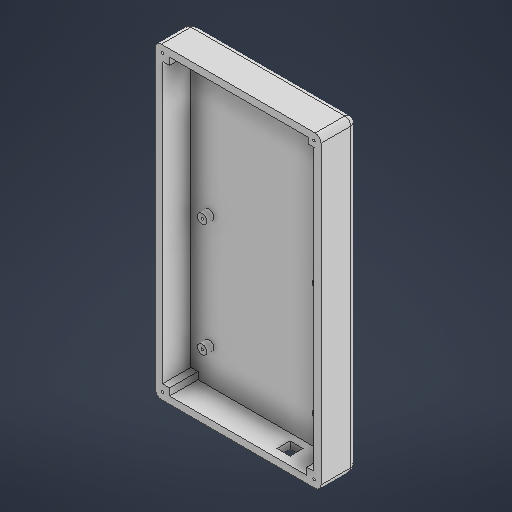
# Autodesk Inventor part: Bottom_Shell
Saved by Autodesk Inventor 2026.2 (Build 302298010, 298A)
## iProperties
Created: 2026-03-03
Part Number: Bottom_Shell
Material: Generic
Document SubType Name: Modeling
Designer: kjedr
Density: 1 g/cm^3
Appearance: Default
Author: kjedr
Autodesk Inventor part; units mm, degrees
ref_plane "YZ Plane" through (0, 0, 0) normal (1, 0, 0) x (0, 1, 0)
ref_plane "XZ Plane" through (0, 0, 0) normal (0, 1, 0) x (-1, 0, 0)
ref_plane "XY Plane" through (0, 0, 0) normal (0, 0, 1) x (1, 0, 0)
sketch "Sketch1" plane through (0, 0, 0) normal (0, 0, 1) x (1, 0, 0)
  line L0 (0, 0) -> (88.9, 0)
  line L1 (88.9, 0) -> (88.9, 165.1)
  line L2 (88.9, 165.1) -> (0, 165.1)
  line L3 (0, 165.1) -> (0, 0)
  dimension "d0" = 88.9
  dimension "d1" = 165.1
  constraints: 8 end point, 2 parallel, 1 horizontal, 1 perpendicular
  measures "d0" distance of L2.end L1.end
  measures "d1" distance of L1.end L0.end
extrude "Extrusion1" add sketch "Sketch1" along normal blind 19.05
sketch "Sketch2" plane through (0, 0, 19.05) normal (0, 0, 1) x (1, 0, 0)
  line L0 (3.81, 3.81) -> (85.09, 3.81)
  line L1 (85.09, 3.81) -> (85.09, 161.29)
  line L2 (85.09, 161.29) -> (3.81, 161.29)
  line L3 (3.81, 161.29) -> (3.81, 3.81)
  line L4 (0, 165.1) -> (0, 0) projected
  line L5 (0, 0) -> (88.9, 0) projected
  line L6 (88.9, 0) -> (88.9, 165.1) projected
  line L7 (88.9, 165.1) -> (0, 165.1) projected
  point P0 (88.9, 82.55)
  dimension "d4" = 3.81
  dimension "d5" = 3.81
  dimension "d6" = 3.81
  dimension "d7" = 3.81
  constraints: 8 end point, 2 parallel, 1 horizontal, 1 midpoint, 1 perpendicular
  measures "d4" distance between parallel lines of L4 L3
  measures "d5" distance between parallel lines of L5 L0
  measures "d6" distance from line of point (88.9, 82.55) L1
  measures "d7" distance between parallel lines of L7 L2
extrude "Extrusion2" cut sketch "Sketch2" against normal blind 15.24 contours L3 L2 L1 L0
fillet "Fillet1" radius 3.175 8 edges at (44.45, 165.1, 0) (88.9, 82.55, 0) (88.9, 0, 9.525) (0, 82.55, 0) (44.45, 0, 0) (88.9, 165.1, 9.525) (0, 165.1, 9.525) (0, 0, 9.525)
sketch "Sketch6" plane through (0, 0, 3.81) normal (0, 0, 1) x (1, 0, 0)
  line L0 (9.181, 90.81) -> (79.719, 90.81) construction
  line L1 (79.719, 90.81) -> (79.719, 6.81) construction
  line L2 (79.719, 6.81) -> (9.181, 6.81) construction
  line L3 (9.181, 6.81) -> (9.181, 90.81) construction
  circle A0 centre (13.6528, 83.516) radius 1.6 construction
  circle A1 centre (75.2732, 83.516) radius 1.6 construction
  circle A2 centre (13.6528, 22.81) radius 1.6 construction
  circle A3 centre (75.2732, 22.81) radius 1.6 construction
  line L4 (3.81, 161.29) -> (85.09, 161.29) projected
  line L5 (3.175, 0) -> (85.725, 0) projected
  line L6 (85.09, 3.81) -> (3.81, 3.81) projected
  circle A4 centre (13.6528, 83.516) radius 2.54
  circle A5 centre (75.2732, 83.516) radius 2.54
  circle A6 centre (13.6528, 22.81) radius 2.54
  circle A7 centre (75.2732, 22.81) radius 2.54
  point P0 (0, 0)
  point P1 (44.45, 90.81)
  point P2 (44.45, 161.29)
  point P3 (18.161, 33.81)
  point P4 (50.719, 19.31)
  point P5 (64.296, 6.81)
  dimension "d18" = 70.538
  dimension "d19" = 84
  dimension "d30" = 3.2
  dimension "d31" = 60.706
  dimension "d32" = 61.6204
  dimension "d33" = 16
  dimension "d34" = 4.4458
  dimension "d36" = 3
  dimension "d37" = 27
  dimension "d38" = 8.98
  dimension "d39" = 12.5
  dimension "d40" = 29
  dimension "d41" = 15.423
  dimension "d69" = 5.08
  dimension "d70" = 5.08
  dimension "d71" = 5.08
  dimension "d72" = 5.08
  constraints: 8 centre point, 8 end point, 4 coincident, 3 equal radius, 3 vertical alignment, 2 horizontal alignment, 2 midpoint, 2 parallel, 1 horizontal, 1 perpendicular, 1 point on line
  measures "d18" distance of L1.end L2.end
  measures "d19" distance of L0.end L1.end
  measures "d30" diameter of A0
  measures "d31" distance of A2.centre A0.centre
  measures "d32" distance of A3.centre A2.centre
  measures "d33" distance from line of L2 A3.centre
  measures "d34" distance from line of L1 A3.centre
  measures "d36" distance between parallel lines of L6 L2
  measures "d37" distance from line of L2 point (18.161, 33.81)
  measures "d38" distance from line of L3 point (18.161, 33.81)
  measures "d39" distance from line of L2 point (50.719, 19.31)
  measures "d40" distance from line of L1 point (50.719, 19.31)
  measures "d41" distance from line of L1 point (64.296, 6.81)
  measures "d69" diameter of A4
  measures "d70" diameter of A5
  measures "d71" diameter of A6
  measures "d72" diameter of A7
sketch "Sketch11" plane through (3.175, 0, 3.175) normal (0, -1, 0) x (1, 0, 0)
  line L0 (85.725, 0) -> (85.725, 15.875) projected
  line L1 (57.6124, 11.4375) -> (64.6124, 11.4375)
  line L2 (64.6124, 11.4375) -> (64.6124, 4.4375)
  line L3 (64.6124, 4.4375) -> (57.6124, 4.4375)
  line L4 (57.6124, 4.4375) -> (57.6124, 11.4375)
  line L5 (57.6124, 11.4375) -> (64.6124, 4.4375) construction
  line L6 (64.6124, 11.4375) -> (57.6124, 4.4375) construction
  line L7 (82.55, 15.875) -> (82.55, 0) projected
  line L8 (0, 15.875) -> (82.55, 15.875) projected
  point P0 (-3.175, -3.175)
  point P1 (61.1124, 7.9375)
  point P2 (64.6124, 7.9375)
  point P3 (82.55, 7.9375)
  point P4 (41.275, 15.875)
  dimension "d43" = 7
  dimension "d44" = 7
  dimension "d68" = 19.8374
  constraints: 12 end point, 5 midpoint, 2 parallel, 1 horizontal, 1 horizontal alignment, 1 perpendicular
  measures "d43" distance of L2.end L3.end
  measures "d44" distance of L1.end L2.end
  measures "d68" horizontal distance of point (41.275, 15.875) point (61.112, 7.938)
extrude "Extrusion5" cut sketch "Sketch11" against normal up to surface (3.81 mm away)
sketch "Sketch12" plane through (0, 0, 3.81) normal (0, 0, 1) x (1, 0, 0)
  line L0 (3.81, 3.81) -> (3.81, 161.29) projected
  line L1 (3.81, 3.81) -> (7.62, 3.81)
  line L2 (7.62, 3.81) -> (7.62, 7.62)
  line L3 (7.62, 7.62) -> (3.81, 7.62)
  line L4 (3.81, 7.62) -> (3.81, 3.81)
  line L5 (3.81, 161.29) -> (85.09, 161.29) projected
  line L6 (3.81, 161.29) -> (7.62, 161.29)
  line L7 (7.62, 161.29) -> (7.62, 157.48)
  line L8 (7.62, 157.48) -> (3.81, 157.48)
  line L9 (3.81, 157.48) -> (3.81, 161.29)
  arc A0 (88.9, 161.925) -> (85.725, 165.1) centre (85.725, 161.925) ccw projected
  line L10 (85.725, 161.925) -> (81.915, 161.925)
  line L11 (81.915, 161.925) -> (81.915, 158.115)
  line L12 (81.915, 158.115) -> (85.725, 158.115)
  line L13 (85.725, 158.115) -> (85.725, 161.925)
  line L14 (85.09, 161.29) -> (85.09, 3.81) projected
  line L15 (85.09, 3.81) -> (81.28, 3.81)
  line L16 (81.28, 3.81) -> (81.28, 7.62)
  line L17 (81.28, 7.62) -> (85.09, 7.62)
  line L18 (85.09, 7.62) -> (85.09, 3.81)
  point P0 (0, 0)
  point P1 (85.09, 158.115)
  point P2 (81.915, 161.29)
  dimension "d47" = 3.81
  dimension "d48" = 3.81
  dimension "d49" = 3.81
  dimension "d50" = 3.81
  dimension "d51" = 3.81
  dimension "d52" = 3.81
  dimension "d53" = 3.81
  dimension "d54" = 3.81
  constraints: 32 end point, 8 parallel, 4 horizontal, 4 perpendicular
  measures "d47" distance of L3.end L2.end
  measures "d48" distance of L2.end L1.end
  measures "d49" distance of L7.end L8.end
  measures "d50" distance of L12.end L11.end
  measures "d51" distance of L11.end L10.end
  measures "d52" distance of L6.end L7.end
  measures "d53" distance of L16.end L17.end
  measures "d54" distance of L15.end L16.end
extrude "Extrusion6" add sketch "Sketch12" along normal up to surface (15.24 mm away) contours L0 L3 L2 L1 | L0 L5 L7 L8 | L5 L14 L12 L11 | L14 L15 L16 L17
sketch "Sketch13" plane through (0, 0, 19.05) normal (0, 0, 1) x (1, 0, 0)
  line L0 (3.81, 7.62) -> (3.81, 157.48) projected
  line L1 (7.62, 161.29) -> (81.915, 161.29) projected
  line L2 (85.09, 158.115) -> (85.09, 7.62) projected
  line L3 (81.28, 3.81) -> (7.62, 3.81) projected
  point P0 (0, 0)
  point P1 (3.81, 161.29)
  point P2 (85.09, 161.29)
  point P3 (85.09, 3.81)
  point P4 (3.81, 3.81)
  dimension "d57" = 0
  dimension "d58" = 0
  dimension "d59" = 0
  dimension "d60" = 0
  constraints: 2 horizontal alignment, 2 vertical alignment
  measures "d57" distance from line of L0 point (3.81, 161.29)
  measures "d58" distance from line of point (3.81, 161.29) L1
  measures "d59" distance from line of point (85.09, 161.29) L2
  measures "d60" distance from line of L3 point (85.09, 3.81)
hole "Hole2" at (3.81, 161.29, 19.05) at (85.09, 161.29, 19.05) at (85.09, 3.81, 19.05) at (3.81, 3.81, 19.05) direction (0, 0, -1) diameter 1.27 end through all
extrude "Extrusion7" add sketch "Sketch6" along normal blind 3.81
sketch "Sketch15" plane through (13.6528, 83.516, 7.62) normal (0, 0, 1) x (1, 0, 0)
  circle A0 centre (0, 0) radius 2.54 projected
  circle A1 centre (61.6204, 0) radius 2.54 projected
  circle A2 centre (61.6204, -60.706) radius 2.54 projected
  circle A3 centre (0, -60.706) radius 2.54 projected
  point P0 (-13.6528, -83.516)
  constraints: 4 coincident
hole "Hole3" at (13.6528, 83.516, 7.62) at (75.2732, 83.516, 7.62) at (75.2732, 22.81, 7.62) at (13.6528, 22.81, 7.62) direction (0, 0, -1) diameter 1.27 depth 6.35
body "Solid1"
